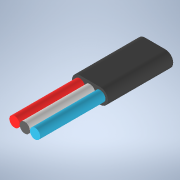
# Autodesk Inventor part: CABLE
Saved by Autodesk Inventor 2022 (Build 260153000, 153)
## iProperties
Created: 2022-07-26
Part Number: CABLE
Material: Generic
Document SubType Name: Modeling
Designer: Nathan Cai
Density: 1 g/cm^3
Appearance: Default
Author: Nathan Cai
Autodesk Inventor part; units mm, degrees
ref_plane "YZ Plane" through (0, 0, 0) normal (1, 0, 0) x (0, 1, 0)
ref_plane "XZ Plane" through (0, 0, 0) normal (0, 1, 0) x (-1, 0, 0)
ref_plane "XY Plane" through (0, 0, 0) normal (0, 0, 1) x (1, 0, 0)
sketch "Sketch1" plane through (0, 0, 0) normal (0, 0, 1) x (1, 0, 0)
  line L0 (-2, 0) -> (2, 0) construction
  line L1 (-2, -1.5) -> (2, -1.5)
  line L2 (2, 1.5) -> (-2, 1.5)
  arc A0 (-2, 1.5) -> (-2, -1.5) centre (-2, 0) ccw
  arc A1 (2, -1.5) -> (2, 1.5) centre (2, 0) ccw
  point P0 (0, 0)
  dimension "d0" = 4
  dimension "d1" = 1.5
  constraints: 8 end point, 4 point on circle, 4 tangent, 2 centre point, 1 horizontal, 1 midpoint, 1 parallel
  measures "d0" distance of L0.start L0.end
  measures "d1" radius of A1
extrude "Extrusion1" add sketch "Sketch1" along normal blind 19.05
sketch "Sketch2" plane through (0, 0, 19.05) normal (0, 0, 1) x (1, 0, 0)
  circle A0 centre (0, 0) radius 1
  circle A1 centre (-2, 0) radius 1
  circle A2 centre (2, 0) radius 1
  line L0 (-2, 0) -> (2, 0)
  point P0 (-1, 0)
  point P1 (1, 0)
  dimension "d4" = 2
  dimension "d5" = 2
  dimension "d6" = 2
  constraints: 3 centre point, 2 end point, 2 equal radius, 1 coincident, 1 horizontal, 1 midpoint
  measures "d4" diameter of A0
  measures "d5" diameter of A1
  measures "d6" diameter of A2
extrude "Extrusion2" add sketch "Sketch2" along normal blind 12.7
body "Solid1"
